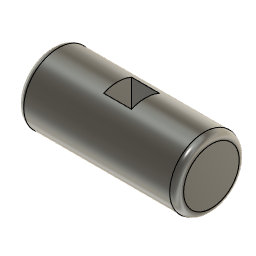
conexão_garra_garra v4 (Autodesk Fusion 360 design; units mm, degrees)
Autodesk Fusion 360 part; units mm, degrees
sketch "Sketch1" plane through (0, 0, 0) normal (1, 0, 0) x (0, 1, 0)
  circle A0 centre (0, 0) radius 5
  circle A1 centre (0, 0) radius 0.5
  dimension "d1" = 10
  dimension "d2" = 1
  constraint coincident A0.centre A1.centre
  constraint concentric A0 A1
  measures "d1" diameter of A0
  measures "d2" diameter of A1
extrude "Extrude1" add sketch "Sketch1" along normal blind 23 contours A0 | A1
extrude "Extrude2" add sketch "Sketch1" against normal blind 1 contours A1
fillet "Fillet1" radius 1 2 edges at (0, -4.6616, -1.8081) (23, -4.6616, -1.8081)
sketch "Sketch2" plane through (0, 0, 0) normal (0, 0, 1) x (1, 0, 0)
  line L0 (0, 15) -> (0, -10) construction
  line L1 (11.5, 15) -> (11.5, -7) construction
  line L2 (-5, 0) -> (27.3814, 0) construction
  line L3 (9.5, 2) -> (13.5, 2)
  line L4 (13.5, 2) -> (13.5, -2)
  line L5 (13.5, -2) -> (9.5, -2)
  line L6 (9.5, -2) -> (9.5, 2)
  line L7 (9.5, 2) -> (13.5, -2) construction
  line L8 (13.5, 2) -> (9.5, -2) construction
  point P0 (11.5, 0)
  dimension "d9" = 11.5
  dimension "d10" = 4
  dimension "d11" = 4
  constraint vertical L0
  constraint vertical L1
  constraint perpendicular L1 L2
  constraint horizontal L3
  constraint perpendicular L3 L4
  constraint parallel L3 L5
  constraint parallel L4 L6
  constraint coincident L7 P0
  constraint coincident L8 P0
  constraint coincident L1 P0
  constraint coincident L2 P0
  measures "d9" distance of L0 L1
  measures "d10" distance of L4.end L5.end
  measures "d11" distance of L3.end L4.end
extrude "Extrude3" cut sketch "Sketch2" along normal blind 5
